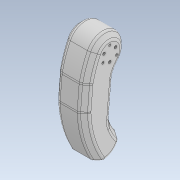
# Autodesk Inventor part: thigh_link
Saved by Autodesk Inventor 2020 (Build 240168000, 168)
## iProperties
Created: 2020-12-22
Part Number: thigh_link
Material: Generic
Document SubType Name: Modeling
Designer: DELL
Density: 1 g/cm^3
Appearance: Default
Author: DELL
Autodesk Inventor part; units mm, degrees
ref_plane "YZ Plane" through (0, 0, 0) normal (1, 0, 0) x (0, 1, 0)
ref_plane "XZ Plane" through (0, 0, 0) normal (0, 1, 0) x (-1, 0, 0)
ref_plane "XY Plane" through (0, 0, 0) normal (0, 0, 1) x (1, 0, 0)
sketch "Sketch1" plane through (0, 0, 0) normal (1, 0, 0) x (0, 1, 0)
  circle A0 centre (0, 0) radius 11.5 construction
  line L0 (0, 0) -> (-120, 0) construction
  circle A1 centre (11.5, 0) radius 1.65
  circle A2 centre (-5.75, 9.959292) radius 1.65
  circle A3 centre (-5.75, -9.959292) radius 1.65
  line L1 (0, 0) -> (-5.75, 9.959292) construction
  line L2 (0, 0) -> (-5.75, -9.959292) construction
  line L3 (0, 11.5) -> (0, -11.5) construction
  circle A4 centre (0, 0) radius 9.715 construction
  circle A5 centre (-9.715, 0) radius 2
  circle A6 centre (4.8575, 8.413437) radius 2
  circle A7 centre (4.8575, -8.413437) radius 2
  line L4 (0, 0) -> (5.75, 9.959292) construction
  line L5 (0, 0) -> (5.75, -9.959292) construction
  circle A8 centre (0, 0) radius 25
  circle A9 centre (-120, 0) radius 20
  circle A10 centre (11.5, 0) radius 2.75
  circle A11 centre (-5.75, 9.959292) radius 2.75
  circle A12 centre (-5.75, -9.959292) radius 2.75
  arc A13 (-60.501798, 37.484969) -> (-22.933883, 34.198203) centre (-54.6875, -112.402301) ccw
  arc A14 (-91.312782, -6.911059) -> (-25.092661, -12.704569) centre (-64.0625, -76.78539) ccw
  line L6 (-25.424583, 34.575363) -> (-57.983444, 37.423894)
  line L7 (-33.741503, -9.868894) -> (-82.302925, -5.62032)
  arc A15 (-22.933883, 34.198203) -> (-25.424583, 34.575363) centre (-27.167698, 14.651469) ccw
  arc A16 (-57.983444, 37.423894) -> (-60.501798, 37.484969) centre (-59.726558, 17.5) ccw
  arc A17 (-25.092661, -12.704569) -> (-33.741503, -9.868894) centre (-35.484618, -29.792788) ccw
  arc A18 (-82.302925, -5.62032) -> (-91.312782, -6.911059) centre (-84.04604, -25.544214) ccw
  line L8 (-130.048077, 17.292662) -> (-108.223684, -16.165345) construction
  arc A19 (-130.048077, 17.292662) -> (-108.223684, -16.165345) centre (-106.542719, 8.778078) ccw
  point P0 (-60, 0)
  point P1 (13, 21.354157)
  point P2 (-13, -21.354157)
  point P3 (-108.223684, -16.165345)
  point P4 (-16.015625, -19.196347)
  point P5 (10.9375, 22.48046)
  point P6 (-130.048077, 17.292662)
  point P7 (-24.212459, 34.469316)
  point P8 (-59.195568, 37.529941)
  point P9 (-29.462766, -10.243235)
  point P10 (-86.581662, -5.245979)
  dimension "d0" = 23
  dimension "d1" = 120
  dimension "d2" = 3.3
  dimension "d3" = 30
  dimension "d4" = 30
  dimension "d5" = 19.43
  dimension "d6" = 4
  dimension "d7" = 30
  dimension "d8" = 50
  dimension "d12" = 5.5
  dimension "d25" = 40
  dimension "d26" = 150
  dimension "d27" = 300
  dimension "d28" = 20
  dimension "d29" = 45
  dimension "d30" = 5
  dimension "d35" = 25
  dimension "d36" = 17.5
  constraints: 27 point on circle, 19 centre point, 18 end point, 12 tangent, 9 equal radius, 7 coincident, 7 point on line, 3 midpoint, 2 horizontal alignment, 1 horizontal, 1 parallel, 1 vertical, 10 other
  measures "d1" distance of L0.end point (0, 0)
  measures "d2" diameter of A1
  measures "d3" angle of L3 L1
  measures "d4" angle of L3 L2
  measures "d5" diameter of A4
  measures "d6" diameter of A6
  measures "d7" angle of L3 L4
  measures "d8" diameter of A8
  measures "d12" diameter of A10
  measures "d25" diameter of A9
  measures "d26" diameter of A14
  measures "d27" diameter of A13
  measures "d28" radius of A15
  measures "d29" distance between parallel lines of L7 L6
  measures "d30" angle of L0 L6
  measures "d35" radius of A19
  measures "d36" distance from line of L0 A16.centre
extrude "Extrusion1" add sketch "Sketch1" against normal mid plane 45 contours A5 | A6 | A7 | A8 | A8 A14 A17 L7 A18 A9 A13 A16 L6 A15 | A9 A19 | A10 | A11 | A12 picked at (-117.802137, -1.737165)
extrude "Extrusion2" cut sketch "Sketch1" along normal blind 35 from surface at -22.5 contours A10 | A11 | A12
extrude "Extrusion3" cut sketch "Sketch1" against normal blind 5 from surface at 22.5 contours A5 | A6 | A7
chamfer "Chamfer1" distance 8 angle 45 1 edges at (22.5, 20.9925, -13.5762)
chamfer "Chamfer2" distance 8 angle 45 1 edges at (-22.5, 20.9925, -13.5762)
fillet "Fillet1" radius 5 12 edges at (-14.5, 20.9925, -13.5762) (-22.5, 14.2749, -9.2318) (14.5, 20.9925, -13.5762) (22.5, 14.2749, -9.2318) (22.5, -127.3662, -5.056) (18.4085, -131.3387, 11.9654) (0, -130.0481, 17.2927) (-18.4085, -131.3387, 11.9654) (-22.5, -127.3662, -5.056) (18.4017, -113.447, -15.2496) (0, -108.2237, -16.1653) (-18.4017, -113.447, -15.2496)
equation "\"d1\" = shank_length"
equation "\"shank_length\" = 120"
body "Solid1"
